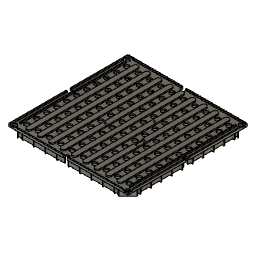
wordclock_Interior_Fusion360 (Autodesk Fusion 360 design; units mm, degrees)
Autodesk Fusion 360 part; units mm, degrees
note: some values were not read from the file. Chosen so that the rebuilt part matches the saved one: which bodies a step acts on.
(part 1 of 3)
sketch "Skizze1" plane through (0, 0, 0) normal (0, 0, 1) x (1, 0, 0)
  line L0 (0, 0) -> (204, 0)
  line L1 (204, 0) -> (204, 204)
  line L2 (204, 204) -> (0, 204)
  line L3 (0, 204) -> (0, 0)
  line L4 (2.15, 201.85) -> (201.85, 201.85)
  line L5 (201.85, 201.85) -> (201.85, 2.15)
  line L6 (201.85, 2.15) -> (2.15, 2.15)
  line L7 (2.15, 2.15) -> (2.15, 201.85)
  line L8 (93.75, 0) -> (100.25, 0)
  line L9 (100.25, 0) -> (100.25, 8.5)
  line L10 (100.25, 8.5) -> (93.75, 8.5)
  line L11 (93.75, 8.5) -> (93.75, 0)
  line L12 (93.75, 204) -> (100.25, 204)
  line L13 (100.25, 204) -> (100.25, 195.5)
  line L14 (100.25, 195.5) -> (93.75, 195.5)
  line L15 (93.75, 195.5) -> (93.75, 204)
  line L16 (0, 105.25) -> (8.5, 105.25)
  line L17 (8.5, 105.25) -> (8.5, 98.75)
  line L18 (8.5, 98.75) -> (0, 98.75)
  line L19 (0, 98.75) -> (0, 105.25)
  line L20 (204, 105.25) -> (195.5, 105.25)
  line L21 (195.5, 105.25) -> (195.5, 98.75)
  line L22 (195.5, 98.75) -> (204, 98.75)
  line L23 (204, 98.75) -> (204, 105.25)
  dimension "d1" = 204
  dimension "d2" = 204
  dimension "d3" = 2.15
  dimension "d4" = 2.15
  dimension "d5" = 2.15
  dimension "d6" = 2.15
  dimension "d387" = 8.5
  dimension "d388" = 6.5
  dimension "d389" = 93.75
  dimension "d390" = 8.5
  dimension "d391" = 6.5
  dimension "d392" = 93.75
  dimension "d397" = 8.5
  dimension "d398" = 6.5
  dimension "d399" = 98.75
  dimension "d415" = 6.5
  dimension "d416" = 8.5
  dimension "d417" = 98.75
  constraint horizontal L0
  constraint vertical L1
  constraint horizontal L2
  constraint vertical L3
  constraint coincident L0.start L3.end
  constraint horizontal L4
  constraint vertical L5
  constraint horizontal L6
  constraint vertical L7
  constraint horizontal L8
  constraint vertical L9
  constraint horizontal L10
  constraint vertical L11
  constraint coincident L0 L8.start
  constraint horizontal L12
  constraint vertical L13
  constraint horizontal L14
  constraint vertical L15
  constraint coincident L2 L12.start
  constraint horizontal L16
  constraint vertical L17
  constraint horizontal L18
  constraint vertical L19
  constraint coincident L3 L16.start
  constraint horizontal L20
  constraint vertical L21
  constraint horizontal L22
  constraint vertical L23
  constraint coincident L1 L20.start
  measures "d1" distance of L0.start L2.end
  measures "d2" distance of L1 L3
  measures "d3" distance of L2 L4
  measures "d4" distance of L1 L5
  measures "d5" distance of L0 L6
  measures "d6" distance of L3 L7
  measures "d387" distance of L8.start L10.end
  measures "d388" distance of L9.end L10.end
  measures "d389" distance of L3 L11
  measures "d390" distance of L12.start L14.end
  measures "d391" distance of L13.end L14.end
  measures "d392" distance of L3 L15
  measures "d397" distance of L16.start L16.end
  measures "d398" distance of L16.end L17.end
  measures "d399" distance of L0 L18
  measures "d415" distance of L20.end L21.end
  measures "d416" distance of L21.end L22.end
  measures "d417" distance of L0 L22
extrude "Extrusion1" add sketch "Skizze1" along normal blind 4 contours L6 L9 L10 L11 | L4 L5 L6 L7 L9 L10 L11 L13 L14 L15 L16 L17 L18 L20 L21 L22 | L7 L16 L17 L18 | L5 L20 L21 L22 | L4 L13 L14 L15 makes body 1
sketch "Skizze2" plane through (0, 0, 0) normal (0, 0, -1) x (1, 0, 0)
  line L0 (201.85, -2.15) -> (2.15, -2.15)
  line L1 (2.15, -2.15) -> (2.15, -201.85)
  line L2 (2.15, -201.85) -> (201.85, -201.85)
  line L3 (201.85, -201.85) -> (201.85, -2.15)
  line L4 (201.85, -18.65) -> (185.35, -2.15)
  line L5 (186.85, -2.15) -> (201.85, -17.15)
  line L6 (201.85, -201.85) -> (201.85, -2.15)
  line L7 (201.85, -2.15) -> (2.15, -2.15)
  line L8 (201.85, -186.85) -> (186.85, -201.85)
  line L9 (201.85, -185.35) -> (185.35, -201.85)
  line L10 (2.15, -186.85) -> (17.15, -201.85)
  line L11 (18.65, -201.85) -> (2.15, -185.35)
  line L12 (18.65, -2.15) -> (2.15, -18.65)
  line L13 (17.15, -2.15) -> (2.15, -17.15)
  point P0 (201.85, -201.85)
  point P1 (2.15, -201.85)
  point P2 (2.15, -2.15)
  point P3 (2.15, -2.15)
  dimension "d9" = 16.5
  dimension "d10" = 16.5
  dimension "d11" = 15
  dimension "d12" = 15
  dimension "d19" = 15
  dimension "d20" = 15
  dimension "d21" = 16.5
  dimension "d22" = 16.5
  dimension "d23" = 16.5
  dimension "d24" = 16.5
  dimension "d25" = 15
  dimension "d26" = 15
  dimension "d27" = 16.5
  dimension "d28" = 16.5
  dimension "d29" = 15
  dimension "d30" = 15
  constraint coincident L3 L4.start
  constraint coincident L0 L4.end
  constraint coincident L0 L5.start
  constraint coincident L3 L5.end
  constraint coincident L3 L8.start
  constraint coincident L2 L8.end
  constraint coincident L3 L9.start
  constraint coincident L2 L9.end
  constraint coincident L1 L10.start
  constraint coincident L2 L10.end
  constraint coincident L2 L11.start
  constraint coincident L1 L11.end
  constraint coincident L0 L12.start
  constraint coincident L1 L12.end
  constraint coincident L0 L13.start
  constraint coincident L1 L13.end
  constraint parallel L12 L13
  measures "d9" distance of L0.start L4.end
  measures "d10" distance of L0.start L4.start
  measures "d11" distance of L0.start L5.start
  measures "d12" distance of L0.start L5.end
  measures "d19" distance of P0 L8.start
  measures "d20" distance of P0 L8.end
  measures "d21" distance of L9.end P0
  measures "d22" distance of L9.start P0
  measures "d23" distance of P1 L11.end
  measures "d24" distance of P1 L11.start
  measures "d25" distance of L10.end P1
  measures "d26" distance of L10.start P1
  measures "d27" distance of L12.start P3
  measures "d28" distance of P3 L12.end
  measures "d29" distance of L13.end P3
  measures "d30" distance of L13.start P3
sketch "Skizze4" plane through (0, 0, 0) normal (0, 0, 1) x (1, 0, 0)
  line L0 (203.9938, 0) -> (0, 0)
  line L1 (0, 203.9937) -> (0, 0)
  line L2 (0, 0) -> (203.9938, 0)
  line L3 (203.9938, 0) -> (203.9938, 203.9937)
  line L4 (203.9938, 203.9937) -> (0, 203.9937)
  line L5 (21.7426, 192.1915) -> (21.7426, 185.9421)
  line L6 (21.7426, 185.9421) -> (20.443, 185.9421)
  line L7 (20.443, 185.9421) -> (20.443, 190.5017)
  line L8 (20.443, 190.5017) -> (17.8837, 190.5017)
  line L9 (17.8837, 190.5017) -> (17.8837, 186.7579)
  line L10 (17.8837, 186.7579) -> (16.5841, 186.7579)
  line L11 (16.5841, 186.7579) -> (16.5841, 190.5017)
  line L12 (16.5841, 190.5017) -> (14.3696, 190.5017)
  line L13 (14.3696, 190.5017) -> (14.3696, 186.0878)
  line L14 (14.3696, 186.0878) -> (13.07, 186.0878)
  line L15 (13.07, 186.0878) -> (13.07, 192.1915)
  line L16 (13.07, 192.1915) -> (21.7426, 192.1915)
  spline S0 degree 3 poles (21.9017, 171.8232) (21.9017, 169.609) (20.7348, 168.298) (19.3291, 168.298) knots 0 0 0 0 1 1 1 1
  spline S1 degree 3 poles (19.3291, 168.298) (18.0693, 168.298) (17.4196, 169.1574) (16.9819, 170.3665) knots 0 0 0 0 1 1 1 1
  line L17 (16.9819, 170.3665) -> (16.4913, 171.6193)
  spline S2 degree 3 poles (16.4913, 171.6193) (16.1863, 172.4788) (15.9343, 173.2508) (15.2713, 173.2508) knots 0 0 0 0 1 1 1 1
  spline S3 degree 3 poles (15.2713, 173.2508) (14.6215, 173.2508) (14.2502, 172.639) (14.2502, 171.7358) knots 0 0 0 0 1 1 1 1
  spline S4 degree 3 poles (14.2502, 171.7358) (14.2502, 170.7744) (14.5287, 170.1043) (14.9928, 169.4633) knots 0 0 0 0 1 1 1 1
  line L18 (14.9928, 169.4633) -> (14.0115, 168.5893)
  spline S5 degree 3 poles (14.0115, 168.5893) (13.3352, 169.3759) (12.9109, 170.483) (12.9109, 171.6484) knots 0 0 0 0 1 1 1 1
  spline S6 degree 3 poles (12.9109, 171.6484) (12.9109, 173.5859) (13.9717, 174.9552) (15.3509, 174.9552) knots 0 0 0 0 1 1 1 1
  spline S7 degree 3 poles (15.3509, 174.9552) (16.6239, 174.9552) (17.3002, 173.9209) (17.6583, 172.9158) knots 0 0 0 0 1 1 1 1
  line L19 (17.6583, 172.9158) -> (18.1754, 171.6193)
  spline S8 degree 3 poles (18.1754, 171.6193) (18.5335, 170.6724) (18.7456, 170.0169) (19.5148, 170.0169) knots 0 0 0 0 1 1 1 1
  spline S9 degree 3 poles (19.5148, 170.0169) (20.1248, 170.0169) (20.5624, 170.6142) (20.5624, 171.7213) knots 0 0 0 0 1 1 1 1
  spline S10 degree 3 poles (20.5624, 171.7213) (20.5624, 172.7264) (20.1646, 173.6733) (19.5811, 174.3871) knots 0 0 0 0 1 1 1 1
  line L20 (19.5811, 174.3871) -> (20.6287, 175.3777)
  spline S11 degree 3 poles (20.6287, 175.3777) (21.4376, 174.4308) (21.9017, 173.1634) (21.9017, 171.8232) knots 0 0 0 0 1 1 1 1
  line L21 (21.7426, 157.5587) -> (21.7426, 155.8397)
  line L22 (21.7426, 155.8397) -> (19.1833, 155.8397)
  line L23 (19.1833, 155.8397) -> (17.6185, 154.485)
  line L24 (17.6185, 154.485) -> (21.7426, 152.0814)
  line L25 (21.7426, 152.0814) -> (21.7426, 150.2022)
  line L26 (21.7426, 150.2022) -> (16.4383, 153.4507)
  line L27 (16.4383, 153.4507) -> (13.07, 150.5081)
  line L28 (13.07, 150.5081) -> (13.07, 152.4019)
  line L29 (13.07, 152.4019) -> (17.0085, 155.796)
  line L30 (17.0085, 155.796) -> (17.0085, 155.8398)
  line L31 (17.0085, 155.8398) -> (13.07, 155.8398)
  line L32 (13.07, 155.8398) -> (13.07, 157.5587)
  line L33 (13.07, 157.5587) -> (21.7426, 157.5587)
  line L34 (21.7426, 140.0602) -> (21.7426, 133.7672)
  line L35 (21.7426, 133.7672) -> (20.443, 133.7672)
  line L36 (20.443, 133.7672) -> (20.443, 136.0688)
  line L37 (20.443, 136.0688) -> (14.3696, 136.0688)
  line L38 (14.3696, 136.0688) -> (14.3696, 133.7672)
  line L39 (14.3696, 133.7672) -> (13.07, 133.7672)
  line L40 (13.07, 133.7672) -> (13.07, 140.0602)
  line L41 (13.07, 140.0602) -> (14.3696, 140.0602)
  line L42 (14.3696, 140.0602) -> (14.3696, 137.7586)
  line L43 (14.3696, 137.7586) -> (20.443, 137.7586)
  line L44 (20.443, 137.7586) -> (20.443, 140.0602)
  line L45 (20.443, 140.0602) -> (21.7426, 140.0602)
  spline S12 degree 3 poles (21.9017, 119.4152) (21.9017, 117.201) (20.7348, 115.8899) (19.3291, 115.8899) knots 0 0 0 0 1 1 1 1
  spline S13 degree 3 poles (19.3291, 115.8899) (18.0693, 115.8899) (17.4196, 116.7494) (16.9819, 117.9585) knots 0 0 0 0 1 1 1 1
  line L46 (16.9819, 117.9585) -> (16.4913, 119.2113)
  spline S14 degree 3 poles (16.4913, 119.2113) (16.1863, 120.0707) (15.9343, 120.8428) (15.2713, 120.8428) knots 0 0 0 0 1 1 1 1
  spline S15 degree 3 poles (15.2713, 120.8428) (14.6215, 120.8428) (14.2502, 120.231) (14.2502, 119.3278) knots 0 0 0 0 1 1 1 1
  spline S16 degree 3 poles (14.2502, 119.3278) (14.2502, 118.3664) (14.5287, 117.6963) (14.9928, 117.0553) knots 0 0 0 0 1 1 1 1
  line L47 (14.9928, 117.0553) -> (14.0115, 116.1813)
  spline S17 degree 3 poles (14.0115, 116.1813) (13.3352, 116.9679) (12.9109, 118.075) (12.9109, 119.2404) knots 0 0 0 0 1 1 1 1
  spline S18 degree 3 poles (12.9109, 119.2404) (12.9109, 121.1779) (13.9717, 122.5472) (15.3509, 122.5472) knots 0 0 0 0 1 1 1 1
  spline S19 degree 3 poles (15.3509, 122.5472) (16.6239, 122.5472) (17.3002, 121.5129) (17.6583, 120.5078) knots 0 0 0 0 1 1 1 1
  line L48 (17.6583, 120.5078) -> (18.1754, 119.2113)
  spline S20 degree 3 poles (18.1754, 119.2113) (18.5335, 118.2644) (18.7456, 117.6089) (19.5148, 117.6089) knots 0 0 0 0 1 1 1 1
  spline S21 degree 3 poles (19.5148, 117.6089) (20.1248, 117.6089) (20.5624, 118.2061) (20.5624, 119.3133) knots 0 0 0 0 1 1 1 1
  spline S22 degree 3 poles (20.5624, 119.3133) (20.5624, 120.3184) (20.1646, 121.2653) (19.5811, 121.9791) knots 0 0 0 0 1 1 1 1
  line L49 (19.5811, 121.9791) -> (20.6287, 122.9696)
  spline S23 degree 3 poles (20.6287, 122.9696) (21.4376, 122.0228) (21.9017, 120.7554) (21.9017, 119.4152) knots 0 0 0 0 1 1 1 1
  line L50 (21.7426, 102.8199) -> (21.7426, 101.1301)
  line L51 (21.7426, 101.1301) -> (14.3696, 101.1301)
  line L52 (14.3696, 101.1301) -> (14.3696, 98.1292)
  line L53 (14.3696, 98.1292) -> (13.07, 98.1292)
  line L54 (13.07, 98.1292) -> (13.07, 105.8207)
  line L55 (13.07, 105.8207) -> (14.3696, 105.8207)
  line L56 (14.3696, 105.8207) -> (14.3696, 102.8199)
  line L57 (14.3696, 102.8199) -> (21.7426, 102.8199)
  spline S24 degree 3 poles (17.1278, 85.4088) (16.2128, 85.1175) (15.2315, 84.8261) (14.2635, 84.5639) knots 0 0 0 0 1 1 1 1
  line L58 (14.2635, 84.5639) -> (14.2635, 84.5056)
  spline S25 degree 3 poles (14.2635, 84.5056) (15.2315, 84.2434) (16.2128, 83.9375) (17.1278, 83.6607) knots 0 0 0 0 1 1 1 1
  line L59 (17.1278, 83.6607) -> (18.1887, 83.3257)
  line L60 (18.1887, 83.3257) -> (18.1887, 85.7439)
  line L61 (18.1887, 85.7439) -> (17.1278, 85.4088)
  line L62 (21.7426, 88.5845) -> (21.7426, 86.8655)
  line L63 (21.7426, 86.8655) -> (19.3954, 86.1226)
  line L64 (19.3954, 86.1226) -> (19.3954, 82.9469)
  line L65 (19.3954, 82.9469) -> (21.7426, 82.2186)
  line L66 (21.7426, 82.2186) -> (21.7426, 80.4268)
  line L67 (21.7426, 80.4268) -> (13.07, 83.5151)
  line L68 (13.07, 83.5151) -> (13.07, 85.4962)
  line L69 (13.07, 85.4962) -> (21.7426, 88.5845)
  line L70 (21.7426, 69.673) -> (21.7426, 67.9832)
  line L71 (21.7426, 67.9832) -> (18.1224, 67.9832)
  line L72 (18.1224, 67.9832) -> (18.1224, 64.2394)
  line L73 (18.1224, 64.2394) -> (16.8228, 64.2394)
  line L74 (16.8228, 64.2394) -> (16.8228, 67.9832)
  line L75 (16.8228, 67.9832) -> (14.3696, 67.9832)
  line L76 (14.3696, 67.9832) -> (14.3696, 63.5839)
  line L77 (14.3696, 63.5839) -> (13.07, 63.5839)
  line L78 (13.07, 63.5839) -> (13.07, 69.673)
  line L79 (13.07, 69.673) -> (21.7426, 69.673)
  spline S26 degree 3 poles (21.9017, 49.5524) (21.9017, 47.4547) (20.8011, 46.2456) (18.4274, 46.2456) knots 0 0 0 0 1 1 1 1
  line L80 (18.4274, 46.2456) -> (13.07, 46.2456)
  line L81 (13.07, 46.2456) -> (13.07, 47.8626)
  line L82 (13.07, 47.8626) -> (18.5467, 47.8626)
  spline S27 degree 3 poles (18.5467, 47.8626) (19.9656, 47.8626) (20.5624, 48.5181) (20.5624, 49.5524) knots 0 0 0 0 1 1 1 1
  spline S28 degree 3 poles (20.5624, 49.5524) (20.5624, 50.5721) (19.9656, 51.1985) (18.5467, 51.1985) knots 0 0 0 0 1 1 1 1
  line L83 (18.5467, 51.1985) -> (13.07, 51.1985)
  line L84 (13.07, 51.1985) -> (13.07, 52.8883)
  line L85 (13.07, 52.8883) -> (18.4274, 52.8883)
  spline S29 degree 3 poles (18.4274, 52.8883) (20.8011, 52.8883) (21.9017, 51.6355) (21.9017, 49.5524) knots 0 0 0 0 1 1 1 1
  spline S30 degree 3 poles (12.3539, 51.0382) (12.3539, 50.5138) (12.0091, 50.1351) (11.5317, 50.1351) knots 0 0 0 0 1 1 1 1
  spline S31 degree 3 poles (11.5317, 50.1351) (11.0544, 50.1351) (10.7096, 50.5138) (10.7096, 51.0382) knots 0 0 0 0 1 1 1 1
  spline S32 degree 3 poles (10.7096, 51.0382) (10.7096, 51.5627) (11.0544, 51.9414) (11.5317, 51.9414) knots 0 0 0 0 1 1 1 1
  spline S33 degree 3 poles (11.5317, 51.9414) (12.0091, 51.9414) (12.3539, 51.5627) (12.3539, 51.0382) knots 0 0 0 0 1 1 1 1
  spline S34 degree 3 poles (12.3539, 48.0956) (12.3539, 47.5712) (12.0091, 47.1925) (11.5317, 47.1925) knots 0 0 0 0 1 1 1 1
  spline S35 degree 3 poles (11.5317, 47.1925) (11.0544, 47.1925) (10.7096, 47.5712) (10.7096, 48.0956) knots 0 0 0 0 1 1 1 1
  spline S36 degree 3 poles (10.7096, 48.0956) (10.7096, 48.6201) (11.0544, 48.9988) (11.5317, 48.9988) knots 0 0 0 0 1 1 1 1
  spline S37 degree 3 poles (11.5317, 48.9988) (12.0091, 48.9988) (12.3539, 48.6201) (12.3539, 48.0956) knots 0 0 0 0 1 1 1 1
  line L86 (21.7426, 35.3898) -> (21.7426, 33.7728)
  line L87 (21.7426, 33.7728) -> (17.95, 33.7728)
  spline S38 degree 3 poles (17.95, 33.7728) (16.9819, 33.7728) (15.9476, 33.9331) (15.0194, 34.0059) knots 0 0 0 0 1 1 1 1
  line L88 (15.0194, 34.0059) -> (15.0194, 33.9622)
  line L89 (15.0194, 33.9622) -> (16.8626, 33.1027)
  line L90 (16.8626, 33.1027) -> (21.7426, 30.5826)
  line L91 (21.7426, 30.5826) -> (21.7426, 28.8054)
  line L92 (21.7426, 28.8054) -> (13.07, 28.8054)
  line L93 (13.07, 28.8054) -> (13.07, 30.4224)
  line L94 (13.07, 30.4224) -> (16.8361, 30.4224)
  spline S39 degree 3 poles (16.8361, 30.4224) (17.8041, 30.4224) (18.9048, 30.2621) (19.7932, 30.1893) knots 0 0 0 0 1 1 1 1
  line L95 (19.7932, 30.1893) -> (19.7932, 30.233)
  line L96 (19.7932, 30.233) -> (17.9367, 31.0925)
  line L97 (17.9367, 31.0925) -> (13.07, 33.6126)
  line L98 (13.07, 33.6126) -> (13.07, 35.3898)
  line L99 (13.07, 35.3898) -> (21.7426, 35.3898)
  line L100 (21.7426, 17.2649) -> (21.7426, 15.5751)
  line L101 (21.7426, 15.5751) -> (18.1224, 15.5751)
  line L102 (18.1224, 15.5751) -> (18.1224, 11.8313)
  line L103 (18.1224, 11.8313) -> (16.8228, 11.8313)
  line L104 (16.8228, 11.8313) -> (16.8228, 15.5751)
  line L105 (16.8228, 15.5751) -> (14.3696, 15.5751)
  line L106 (14.3696, 15.5751) -> (14.3696, 11.1758)
  line L107 (14.3696, 11.1758) -> (13.07, 11.1758)
  line L108 (13.07, 11.1758) -> (13.07, 17.2649)
  line L109 (13.07, 17.2649) -> (21.7426, 17.2649)
  line L110 (40.7851, 192.8033) -> (40.7851, 185.7819)
  line L111 (40.7851, 185.7819) -> (39.4855, 185.7819)
  line L112 (39.4855, 185.7819) -> (39.4855, 190.7347)
  line L113 (39.4855, 190.7347) -> (33.0408, 185.8401)
  line L114 (33.0408, 185.8401) -> (32.1125, 185.8401)
  line L115 (32.1125, 185.8401) -> (32.1125, 192.3663)
  line L116 (32.1125, 192.3663) -> (33.3988, 192.3663)
  line L117 (33.3988, 192.3663) -> (33.3988, 187.9232)
  line L118 (33.3988, 187.9232) -> (39.8568, 192.8033)
  line L119 (39.8568, 192.8033) -> (40.7851, 192.8033)
  line L120 (40.7851, 174.7221) -> (40.7851, 168.4728)
  line L121 (40.7851, 168.4728) -> (39.4855, 168.4728)
  line L122 (39.4855, 168.4728) -> (39.4855, 173.0323)
  line L123 (39.4855, 173.0323) -> (36.9262, 173.0323)
  line L124 (36.9262, 173.0323) -> (36.9262, 169.2885)
  line L125 (36.9262, 169.2885) -> (35.6266, 169.2885)
  line L126 (35.6266, 169.2885) -> (35.6266, 173.0323)
  line L127 (35.6266, 173.0323) -> (33.4121, 173.0323)
  line L128 (33.4121, 173.0323) -> (33.4121, 168.6184)
  line L129 (33.4121, 168.6184) -> (32.1125, 168.6184)
  line L130 (32.1125, 168.6184) -> (32.1125, 174.7221)
  line L131 (32.1125, 174.7221) -> (40.7851, 174.7221)
  line L132 (40.7851, 157.7044) -> (40.7851, 156.0146)
  line L133 (40.7851, 156.0146) -> (36.9394, 156.0146)
  line L134 (36.9394, 156.0146) -> (36.9394, 152.7515)
  line L135 (36.9394, 152.7515) -> (40.7851, 152.7515)
  line L136 (40.7851, 152.7515) -> (40.7851, 151.0617)
  line L137 (40.7851, 151.0617) -> (32.1125, 151.0617)
  line L138 (32.1125, 151.0617) -> (32.1125, 152.7515)
  line L139 (32.1125, 152.7515) -> (35.6001, 152.7515)
  line L140 (35.6001, 152.7515) -> (35.6001, 156.0146)
  line L141 (35.6001, 156.0146) -> (32.1125, 156.0146)
  line L142 (32.1125, 156.0146) -> (32.1125, 157.7044)
  line L143 (32.1125, 157.7044) -> (40.7851, 157.7044)
  line L144 (40.7851, 140.2059) -> (40.7851, 138.5889)
  line L145 (40.7851, 138.5889) -> (36.9925, 138.5889)
  spline S40 degree 3 poles (36.9925, 138.5889) (36.0244, 138.5889) (34.9901, 138.7492) (34.0618, 138.822) knots 0 0 0 0 1 1 1 1
  line L146 (34.0618, 138.822) -> (34.0618, 138.7783)
  line L147 (34.0618, 138.7783) -> (35.9051, 137.9188)
  line L148 (35.9051, 137.9188) -> (40.7851, 135.3987)
  line L149 (40.7851, 135.3987) -> (40.7851, 133.6215)
  line L150 (40.7851, 133.6215) -> (32.1125, 133.6215)
  line L151 (32.1125, 133.6215) -> (32.1125, 135.2384)
  line L152 (32.1125, 135.2384) -> (35.8786, 135.2384)
  spline S41 degree 3 poles (35.8786, 135.2384) (36.8466, 135.2384) (37.9473, 135.0782) (38.8357, 135.0054) knots 0 0 0 0 1 1 1 1
  line L153 (38.8357, 135.0054) -> (38.8357, 135.0491)
  line L154 (38.8357, 135.0491) -> (36.9792, 135.9085)
  line L155 (36.9792, 135.9085) -> (32.1125, 138.4287)
  line L156 (32.1125, 138.4287) -> (32.1125, 140.2059)
  line L157 (32.1125, 140.2059) -> (40.7851, 140.2059)
  line L158 (40.7851, 122.9259) -> (40.7851, 115.9045)
  line L159 (40.7851, 115.9045) -> (39.4855, 115.9045)
  line L160 (39.4855, 115.9045) -> (39.4855, 120.8574)
  line L161 (39.4855, 120.8574) -> (33.0408, 115.9628)
  line L162 (33.0408, 115.9628) -> (32.1125, 115.9628)
  line L163 (32.1125, 115.9628) -> (32.1125, 122.4889)
  line L164 (32.1125, 122.4889) -> (33.3988, 122.4889)
  line L165 (33.3988, 122.4889) -> (33.3988, 118.0459)
  line L166 (33.3988, 118.0459) -> (39.8568, 122.9259)
  line L167 (39.8568, 122.9259) -> (40.7851, 122.9259)
  line L168 (40.7851, 104.8884) -> (40.7851, 103.0093)
  line L169 (40.7851, 103.0093) -> (37.7086, 102.2809)
  spline S42 degree 3 poles (37.7086, 102.2809) (37.1649, 102.1498) (36.6212, 102.077) (36.0907, 101.9895) knots 0 0 0 0 1 1 1 1
  line L170 (36.0907, 101.9895) -> (36.0907, 101.9458)
  spline S43 degree 3 poles (36.0907, 101.9458) (36.6212, 101.8876) (37.1649, 101.771) (37.7086, 101.6399) knots 0 0 0 0 1 1 1 1
  line L171 (37.7086, 101.6399) -> (40.7851, 100.897)
  line L172 (40.7851, 100.897) -> (40.7851, 98.9887)
  line L173 (40.7851, 98.9887) -> (32.1125, 97.7067)
  line L174 (32.1125, 97.7067) -> (32.1125, 99.4111)
  line L175 (32.1125, 99.4111) -> (37.1383, 99.8773)
  spline S44 degree 3 poles (37.1383, 99.8773) (37.8544, 99.9355) (38.3981, 99.9501) (39.2203, 99.9938) knots 0 0 0 0 1 1 1 1
  line L176 (39.2203, 99.9938) -> (39.2203, 100.0521)
  spline S45 degree 3 poles (39.2203, 100.0521) (38.3981, 100.1978) (37.8544, 100.3289) (37.1383, 100.5182) knots 0 0 0 0 1 1 1 1
  line L177 (37.1383, 100.5182) -> (34.327, 101.2612)
  line L178 (34.327, 101.2612) -> (34.327, 102.5285)
  line L179 (34.327, 102.5285) -> (37.1383, 103.3152)
  spline S46 degree 3 poles (37.1383, 103.3152) (37.8677, 103.49) (38.4114, 103.6211) (39.2203, 103.7813) knots 0 0 0 0 1 1 1 1
  line L180 (39.2203, 103.7813) -> (39.2203, 103.825)
  spline S47 degree 3 poles (39.2203, 103.825) (38.4114, 103.8541) (37.8677, 103.8978) (37.1383, 103.9561) knots 0 0 0 0 1 1 1 1
  line L181 (37.1383, 103.9561) -> (32.1125, 104.4368)
  line L182 (32.1125, 104.4368) -> (32.1125, 106.2432)
  line L183 (32.1125, 106.2432) -> (40.7851, 104.8884)
  spline S48 degree 3 poles (36.1703, 85.4088) (35.2553, 85.1175) (34.274, 84.8261) (33.306, 84.5639) knots 0 0 0 0 1 1 1 1
  line L184 (33.306, 84.5639) -> (33.306, 84.5056)
  spline S49 degree 3 poles (33.306, 84.5056) (34.274, 84.2434) (35.2553, 83.9375) (36.1703, 83.6607) knots 0 0 0 0 1 1 1 1
  line L185 (36.1703, 83.6607) -> (37.2312, 83.3257)
  line L186 (37.2312, 83.3257) -> (37.2312, 85.7439)
  line L187 (37.2312, 85.7439) -> (36.1703, 85.4088)
  line L188 (40.7851, 88.5845) -> (40.7851, 86.8655)
  line L189 (40.7851, 86.8655) -> (38.4379, 86.1226)
  line L190 (38.4379, 86.1226) -> (38.4379, 82.9469)
  line L191 (38.4379, 82.9469) -> (40.7851, 82.2186)
  line L192 (40.7851, 82.2186) -> (40.7851, 80.4268)
  line L193 (40.7851, 80.4268) -> (32.1125, 83.5151)
  line L194 (32.1125, 83.5151) -> (32.1125, 85.4962)
  line L195 (32.1125, 85.4962) -> (40.7851, 88.5845)
  line L196 (40.7851, 70.3285) -> (40.7851, 68.7116)
  line L197 (40.7851, 68.7116) -> (36.9925, 68.7116)
  spline S50 degree 3 poles (36.9925, 68.7116) (36.0244, 68.7116) (34.9901, 68.8718) (34.0618, 68.9446) knots 0 0 0 0 1 1 1 1
  line L198 (34.0618, 68.9446) -> (34.0618, 68.9009)
  line L199 (34.0618, 68.9009) -> (35.9051, 68.0415)
  line L200 (35.9051, 68.0415) -> (40.7851, 65.5213)
  line L201 (40.7851, 65.5213) -> (40.7851, 63.7441)
  line L202 (40.7851, 63.7441) -> (32.1125, 63.7441)
  line L203 (32.1125, 63.7441) -> (32.1125, 65.3611)
  line L204 (32.1125, 65.3611) -> (35.8786, 65.3611)
  spline S51 degree 3 poles (35.8786, 65.3611) (36.8466, 65.3611) (37.9473, 65.2008) (38.8357, 65.128) knots 0 0 0 0 1 1 1 1
  line L205 (38.8357, 65.128) -> (38.8357, 65.1717)
  line L206 (38.8357, 65.1717) -> (36.9792, 66.0312)
  line L207 (36.9792, 66.0312) -> (32.1125, 68.5513)
  line L208 (32.1125, 68.5513) -> (32.1125, 70.3285)
  line L209 (32.1125, 70.3285) -> (40.7851, 70.3285)
  line L210 (40.7851, 53.0485) -> (40.7851, 46.0271)
  line L211 (40.7851, 46.0271) -> (39.4855, 46.0271)
  line L212 (39.4855, 46.0271) -> (39.4855, 50.98)
  line L213 (39.4855, 50.98) -> (33.0408, 46.0854)
  line L214 (33.0408, 46.0854) -> (32.1125, 46.0854)
  line L215 (32.1125, 46.0854) -> (32.1125, 52.6115)
  line L216 (32.1125, 52.6115) -> (33.3988, 52.6115)
  line L217 (33.3988, 52.6115) -> (33.3988, 48.1685)
  line L218 (33.3988, 48.1685) -> (39.8568, 53.0485)
  line L219 (39.8568, 53.0485) -> (40.7851, 53.0485)
  line L220 (40.7851, 35.2441) -> (40.7851, 28.9511)
  line L221 (40.7851, 28.9511) -> (39.4855, 28.9511)
  line L222 (39.4855, 28.9511) -> (39.4855, 31.2527)
  line L223 (39.4855, 31.2527) -> (33.4121, 31.2527)
  line L224 (33.4121, 31.2527) -> (33.4121, 28.9511)
  line L225 (33.4121, 28.9511) -> (32.1125, 28.9511)
  line L226 (32.1125, 28.9511) -> (32.1125, 35.2441)
  line L227 (32.1125, 35.2441) -> (33.4121, 35.2441)
  line L228 (33.4121, 35.2441) -> (33.4121, 32.9425)
  line L229 (33.4121, 32.9425) -> (39.4855, 32.9425)
  line L230 (39.4855, 32.9425) -> (39.4855, 35.2441)
  line L231 (39.4855, 35.2441) -> (40.7851, 35.2441)
  spline S52 degree 3 poles (40.9442, 14.0456) (40.9442, 12.8219) (40.4668, 11.7439) (39.9099, 11.1321) knots 0 0 0 0 1 1 1 1
  line L232 (39.9099, 11.1321) -> (36.0907, 11.1321)
  line L233 (36.0907, 11.1321) -> (36.0907, 14.3078)
  line L234 (36.0907, 14.3078) -> (37.3505, 14.3078)
  line L235 (37.3505, 14.3078) -> (37.3505, 12.6617)
  line L236 (37.3505, 12.6617) -> (39.2203, 12.6617)
  spline S53 degree 3 poles (39.2203, 12.6617) (39.4723, 12.9385) (39.6049, 13.4338) (39.6049, 13.9436) knots 0 0 0 0 1 1 1 1
  spline S54 degree 3 poles (39.6049, 13.9436) (39.6049, 15.6334) (38.4114, 16.5511) (36.4355, 16.5511) knots 0 0 0 0 1 1 1 1
  spline S55 degree 3 poles (36.4355, 16.5511) (34.4862, 16.5511) (33.2927, 15.4877) (33.2927, 13.9728) knots 0 0 0 0 1 1 1 1
  spline S56 degree 3 poles (33.2927, 13.9728) (33.2927, 13.1424) (33.5844, 12.6471) (33.9955, 12.2101) knots 0 0 0 0 1 1 1 1
  line L237 (33.9955, 12.2101) -> (33.0408, 11.2778)
  spline S57 degree 3 poles (33.0408, 11.2778) (32.4971, 11.8459) (31.9534, 12.7054) (31.9534, 13.9728) knots 0 0 0 0 1 1 1 1
  spline S58 degree 3 poles (31.9534, 13.9728) (31.9534, 16.4492) (33.6242, 18.2992) (36.4753, 18.2992) knots 0 0 0 0 1 1 1 1
  spline S59 degree 3 poles (36.4753, 18.2992) (39.3529, 18.2992) (40.9442, 16.4637) (40.9442, 14.0456) knots 0 0 0 0 1 1 1 1
  line L238 (59.8276, 192.5556) -> (59.8276, 189.9627)
  spline S60 degree 3 poles (59.8276, 189.9627) (59.8276, 187.2386) (58.3291, 185.5634) (55.4515, 185.5634) knots 0 0 0 0 1 1 1 1
  spline S61 degree 3 poles (55.4515, 185.5634) (52.5872, 185.5634) (51.155, 187.2386) (51.155, 190.0501) knots 0 0 0 0 1 1 1 1
  line L239 (51.155, 190.0501) -> (51.155, 192.5556)
  line L240 (51.155, 192.5556) -> (59.8276, 192.5556)
  line L241 (58.5811, 190.8658) -> (52.4015, 190.8658)
  line L242 (52.4015, 190.8658) -> (52.4015, 190.152)
  spline S62 degree 3 poles (52.4015, 190.152) (52.4015, 188.3311) (53.3298, 187.2969) (55.4515, 187.2969) knots 0 0 0 0 1 1 1 1
  spline S63 degree 3 poles (55.4515, 187.2969) (57.5865, 187.2969) (58.5811, 188.3311) (58.5811, 190.152) knots 0 0 0 0 1 1 1 1
  line L243 (58.5811, 190.152) -> (58.5811, 190.8658)
  line L244 (59.8276, 174.9989) -> (59.8276, 173.3091)
  line L245 (59.8276, 173.3091) -> (56.4328, 173.3091)
  line L246 (56.4328, 173.3091) -> (56.4328, 171.8815)
  line L247 (56.4328, 171.8815) -> (59.8276, 169.8421)
  line L248 (59.8276, 169.8421) -> (59.8276, 167.9338)
  line L249 (59.8276, 167.9338) -> (56.2074, 170.2063)
  spline S64 degree 3 poles (56.2074, 170.2063) (55.8493, 169.07) (55.0404, 168.3125) (53.7276, 168.3125) knots 0 0 0 0 1 1 1 1
  spline S65 degree 3 poles (53.7276, 168.3125) (51.7915, 168.3125) (51.155, 169.8421) (51.155, 171.8232) knots 0 0 0 0 1 1 1 1
  line L250 (51.155, 171.8232) -> (51.155, 174.9989)
  line L251 (51.155, 174.9989) -> (59.8276, 174.9989)
  line L252 (55.2128, 173.3091) -> (52.3883, 173.3091)
  line L253 (52.3883, 173.3091) -> (52.3883, 171.998)
  spline S66 degree 3 poles (52.3883, 171.998) (52.3883, 170.687) (52.733, 169.9732) (53.7276, 169.9732) knots 0 0 0 0 1 1 1 1
  spline S67 degree 3 poles (53.7276, 169.9732) (54.7089, 169.9732) (55.2128, 170.687) (55.2128, 171.998) knots 0 0 0 0 1 1 1 1
  line L254 (55.2128, 171.998) -> (55.2128, 173.3091)
  line L255 (59.8276, 157.2528) -> (59.8276, 151.0034)
  line L256 (59.8276, 151.0034) -> (58.528, 151.0034)
  line L257 (58.528, 151.0034) -> (58.528, 155.563)
  line L258 (58.528, 155.563) -> (55.9687, 155.563)
  line L259 (55.9687, 155.563) -> (55.9687, 151.8192)
  line L260 (55.9687, 151.8192) -> (54.6691, 151.8192)
  line L261 (54.6691, 151.8192) -> (54.6691, 155.563)
  line L262 (54.6691, 155.563) -> (52.4545, 155.563)
  line L263 (52.4545, 155.563) -> (52.4545, 151.1491)
  line L264 (52.4545, 151.1491) -> (51.155, 151.1491)
  line L265 (51.155, 151.1491) -> (51.155, 157.2528)
  line L266 (51.155, 157.2528) -> (59.8276, 157.2528)
  line L267 (59.8276, 140.0602) -> (59.8276, 133.7672)
  line L268 (59.8276, 133.7672) -> (58.528, 133.7672)
  line L269 (58.528, 133.7672) -> (58.528, 136.0688)
  line L270 (58.528, 136.0688) -> (52.4545, 136.0688)
  line L271 (52.4545, 136.0688) -> (52.4545, 133.7672)
  line L272 (52.4545, 133.7672) -> (51.155, 133.7672)
  line L273 (51.155, 133.7672) -> (51.155, 140.0602)
  line L274 (51.155, 140.0602) -> (52.4545, 140.0602)
  line L275 (52.4545, 140.0602) -> (52.4545, 137.7586)
  line L276 (52.4545, 137.7586) -> (58.528, 137.7586)
  line L277 (58.528, 137.7586) -> (58.528, 140.0602)
  line L278 (58.528, 140.0602) -> (59.8276, 140.0602)
  line L279 (59.8276, 120.4349) -> (59.8276, 118.4392)
  line L280 (59.8276, 118.4392) -> (51.155, 115.482)
  line L281 (51.155, 115.482) -> (51.155, 117.2155)
  line L282 (51.155, 117.2155) -> (55.5178, 118.5412)
  spline S68 degree 3 poles (55.5178, 118.5412) (56.4991, 118.8325) (57.3478, 119.051) (58.3424, 119.3715) knots 0 0 0 0 1 1 1 1
  line L283 (58.3424, 119.3715) -> (58.3424, 119.4298)
  spline S69 degree 3 poles (58.3424, 119.4298) (57.3478, 119.7502) (56.4991, 119.9688) (55.5178, 120.2747) knots 0 0 0 0 1 1 1 1
  line L284 (55.5178, 120.2747) -> (51.155, 121.6149)
  line L285 (51.155, 121.6149) -> (51.155, 123.4066)
  line L286 (51.155, 123.4066) -> (59.8276, 120.4349)
  line L287 (59.8276, 105.1215) -> (59.8276, 98.8285)
  line L288 (59.8276, 98.8285) -> (58.528, 98.8285)
  line L289 (58.528, 98.8285) -> (58.528, 101.1301)
  line L290 (58.528, 101.1301) -> (52.4545, 101.1301)
  line L291 (52.4545, 101.1301) -> (52.4545, 98.8285)
  line L292 (52.4545, 98.8285) -> (51.155, 98.8285)
  line L293 (51.155, 98.8285) -> (51.155, 105.1215)
  line L294 (51.155, 105.1215) -> (52.4545, 105.1215)
  line L295 (52.4545, 105.1215) -> (52.4545, 102.8199)
  line L296 (52.4545, 102.8199) -> (58.528, 102.8199)
  line L297 (58.528, 102.8199) -> (58.528, 105.1215)
  line L298 (58.528, 105.1215) -> (59.8276, 105.1215)
  line L299 (59.8276, 87.3754) -> (59.8276, 81.1261)
  line L300 (59.8276, 81.1261) -> (58.528, 81.1261)
  line L301 (58.528, 81.1261) -> (58.528, 85.6856)
  line L302 (58.528, 85.6856) -> (55.9687, 85.6856)
  line L303 (55.9687, 85.6856) -> (55.9687, 81.9418)
  line L304 (55.9687, 81.9418) -> (54.6691, 81.9418)
  line L305 (54.6691, 81.9418) -> (54.6691, 85.6856)
  line L306 (54.6691, 85.6856) -> (52.4545, 85.6856)
  line L307 (52.4545, 85.6856) -> (52.4545, 81.2717)
  line L308 (52.4545, 81.2717) -> (51.155, 81.2717)
  line L309 (51.155, 81.2717) -> (51.155, 87.3754)
  line L310 (51.155, 87.3754) -> (59.8276, 87.3754)
  line L311 (59.8276, 70.1828) -> (59.8276, 68.493)
  line L312 (59.8276, 68.493) -> (56.4328, 68.493)
  line L313 (56.4328, 68.493) -> (56.4328, 67.0655)
  line L314 (56.4328, 67.0655) -> (59.8276, 65.026)
  line L315 (59.8276, 65.026) -> (59.8276, 63.1177)
  line L316 (59.8276, 63.1177) -> (56.2074, 65.3902)
  spline S70 degree 3 poles (56.2074, 65.3902) (55.8493, 64.254) (55.0404, 63.4965) (53.7276, 63.4965) knots 0 0 0 0 1 1 1 1
  spline S71 degree 3 poles (53.7276, 63.4965) (51.7915, 63.4965) (51.155, 65.026) (51.155, 67.0072) knots 0 0 0 0 1 1 1 1
  line L317 (51.155, 67.0072) -> (51.155, 70.1829)
  line L318 (51.155, 70.1829) -> (59.8276, 70.1828)
  line L319 (55.2128, 68.493) -> (52.3883, 68.493)
  line L320 (52.3883, 68.493) -> (52.3883, 67.182)
  spline S72 degree 3 poles (52.3883, 67.182) (52.3883, 65.8709) (52.733, 65.1571) (53.7276, 65.1571) knots 0 0 0 0 1 1 1 1
  spline S73 degree 3 poles (53.7276, 65.1571) (54.7089, 65.1571) (55.2128, 65.8709) (55.2128, 67.182) knots 0 0 0 0 1 1 1 1
  line L321 (55.2128, 67.182) -> (55.2128, 68.493)
  line L322 (59.8276, 50.4119) -> (59.8276, 48.7221)
  line L323 (59.8276, 48.7221) -> (52.4546, 48.7221)
  line L324 (52.4546, 48.7221) -> (52.4546, 45.7212)
  line L325 (52.4546, 45.7212) -> (51.155, 45.7212)
  line L326 (51.155, 45.7212) -> (51.155, 53.4128)
  line L327 (51.155, 53.4128) -> (52.4546, 53.4128)
  line L328 (52.4546, 53.4128) -> (52.4546, 50.4119)
  line L329 (52.4546, 50.4119) -> (59.8276, 50.4119)
  line L330 (59.8276, 34.9674) -> (59.8276, 28.718)
  line L331 (59.8276, 28.718) -> (58.528, 28.718)
  line L332 (58.528, 28.718) -> (58.528, 33.2775)
  line L333 (58.528, 33.2775) -> (55.9687, 33.2775)
  line L334 (55.9687, 33.2775) -> (55.9687, 29.5337)
  line L335 (55.9687, 29.5337) -> (54.6691, 29.5337)
  line L336 (54.6691, 29.5337) -> (54.6691, 33.2775)
  line L337 (54.6691, 33.2775) -> (52.4545, 33.2775)
  line L338 (52.4545, 33.2775) -> (52.4545, 28.8637)
  line L339 (52.4545, 28.8637) -> (51.155, 28.8637)
  line L340 (51.155, 28.8637) -> (51.155, 34.9674)
  line L341 (51.155, 34.9674) -> (59.8276, 34.9674)
  line L342 (59.8276, 17.2504) -> (59.8276, 11.103)
  line L343 (59.8276, 11.103) -> (58.528, 11.103)
  line L344 (58.528, 11.103) -> (58.528, 15.5752)
  line L345 (58.528, 15.5752) -> (51.155, 15.5752)
  line L346 (51.155, 15.5752) -> (51.155, 17.2504)
  line L347 (51.155, 17.2504) -> (59.8276, 17.2504)
  line L348 (78.8701, 190.3123) -> (78.8701, 188.3166)
  line L349 (78.8701, 188.3166) -> (70.1975, 185.3594)
  line L350 (70.1975, 185.3594) -> (70.1975, 187.0929)
  line L351 (70.1975, 187.0929) -> (74.5603, 188.4185)
  spline S74 degree 3 poles (74.5603, 188.4185) (75.5416, 188.7099) (76.3903, 188.9284) (77.3849, 189.2489) knots 0 0 0 0 1 1 1 1
  line L352 (77.3849, 189.2489) -> (77.3849, 189.3071)
  spline S75 degree 3 poles (77.3849, 189.3071) (76.3903, 189.6276) (75.5416, 189.8461) (74.5603, 190.152) knots 0 0 0 0 1 1 1 1
  line L353 (74.5603, 190.152) -> (70.1975, 191.4922)
  line L354 (70.1975, 191.4922) -> (70.1975, 193.284)
  line L355 (70.1975, 193.284) -> (78.8701, 190.3123)
  spline S76 degree 3 poles (79.0292, 171.8524) (79.0292, 169.6381) (77.3981, 168.1086) (74.494, 168.1086) knots 0 0 0 0 1 1 1 1
  spline S77 degree 3 poles (74.494, 168.1086) (71.6429, 168.1086) (70.0384, 169.6381) (70.0384, 171.8524) knots 0 0 0 0 1 1 1 1
  spline S78 degree 3 poles (70.0384, 171.8524) (70.0384, 174.0666) (71.6429, 175.5962) (74.494, 175.5962) knots 0 0 0 0 1 1 1 1
  spline S79 degree 3 poles (74.494, 175.5962) (77.3981, 175.5962) (79.0292, 174.0666) (79.0292, 171.8524) knots 0 0 0 0 1 1 1 1
  spline S80 degree 3 poles (77.6899, 171.8524) (77.6899, 173.076) (76.5362, 173.8626) (74.494, 173.8626) knots 0 0 0 0 1 1 1 1
  spline S81 degree 3 poles (74.494, 173.8626) (72.5049, 173.8626) (71.3777, 173.076) (71.3777, 171.8524) knots 0 0 0 0 1 1 1 1
  spline S82 degree 3 poles (71.3777, 171.8524) (71.3777, 170.6287) (72.5049, 169.8421) (74.494, 169.8421) knots 0 0 0 0 1 1 1 1
  spline S83 degree 3 poles (74.494, 169.8421) (76.5362, 169.8421) (77.6899, 170.6287) (77.6899, 171.8524) knots 0 0 0 0 1 1 1 1
  line L356 (78.8701, 157.5296) -> (78.8701, 155.8398)
  line L357 (78.8701, 155.8398) -> (75.4753, 155.8398)
  line L358 (75.4753, 155.8398) -> (75.4753, 154.4122)
  line L359 (75.4753, 154.4122) -> (78.8701, 152.3728)
  line L360 (78.8701, 152.3728) -> (78.8701, 150.4644)
  line L361 (78.8701, 150.4644) -> (75.2499, 152.7369)
  spline S84 degree 3 poles (75.2499, 152.7369) (74.8918, 151.6007) (74.0829, 150.8432) (72.7701, 150.8432) knots 0 0 0 0 1 1 1 1
  spline S85 degree 3 poles (72.7701, 150.8432) (70.834, 150.8432) (70.1975, 152.3728) (70.1975, 154.3539) knots 0 0 0 0 1 1 1 1
  line L362 (70.1975, 154.3539) -> (70.1975, 157.5296)
  line L363 (70.1975, 157.5296) -> (78.8701, 157.5296)
  line L364 (74.2553, 155.8398) -> (71.4307, 155.8398)
  line L365 (71.4307, 155.8398) -> (71.4307, 154.5287)
  spline S86 degree 3 poles (71.4307, 154.5287) (71.4307, 153.2177) (71.7755, 152.5039) (72.7701, 152.5039) knots 0 0 0 0 1 1 1 1
  spline S87 degree 3 poles (72.7701, 152.5039) (73.7514, 152.5039) (74.2553, 153.2177) (74.2553, 154.5287) knots 0 0 0 0 1 1 1 1
  line L366 (74.2553, 154.5287) -> (74.2553, 155.8398)
  line L367 (78.8701, 139.5504) -> (78.8701, 137.8605)
  line L368 (78.8701, 137.8605) -> (75.2499, 137.8605)
  line L369 (75.2499, 137.8605) -> (75.2499, 134.1168)
  line L370 (75.2499, 134.1168) -> (73.9503, 134.1168)
  line L371 (73.9503, 134.1168) -> (73.9503, 137.8605)
  line L372 (73.9503, 137.8605) -> (71.4971, 137.8605)
  line L373 (71.4971, 137.8605) -> (71.4971, 133.4612)
  line L374 (71.4971, 133.4612) -> (70.1975, 133.4612)
  line L375 (70.1975, 133.4612) -> (70.1975, 139.5504)
  line L376 (70.1975, 139.5504) -> (78.8701, 139.5504)
  spline S88 degree 3 poles (79.0292, 119.4298) (79.0292, 117.3321) (77.9286, 116.123) (75.5549, 116.123) knots 0 0 0 0 1 1 1 1
  line L377 (75.5549, 116.123) -> (70.1975, 116.123)
  line L378 (70.1975, 116.123) -> (70.1975, 117.74)
  line L379 (70.1975, 117.74) -> (75.6742, 117.74)
  spline S89 degree 3 poles (75.6742, 117.74) (77.0931, 117.74) (77.6899, 118.3955) (77.6899, 119.4297) knots 0 0 0 0 1 1 1 1
  spline S90 degree 3 poles (77.6899, 119.4297) (77.6899, 120.4495) (77.0931, 121.0759) (75.6742, 121.0759) knots 0 0 0 0 1 1 1 1
  line L380 (75.6742, 121.0759) -> (70.1975, 121.0759)
  line L381 (70.1975, 121.0759) -> (70.1975, 122.7656)
  line L382 (70.1975, 122.7656) -> (75.5549, 122.7656)
  spline S91 degree 3 poles (75.5549, 122.7656) (77.9286, 122.7656) (79.0292, 121.5129) (79.0292, 119.4298) knots 0 0 0 0 1 1 1 1
  line L383 (78.8701, 105.2672) -> (78.8701, 103.6502)
  line L384 (78.8701, 103.6502) -> (75.0775, 103.6502)
  spline S92 degree 3 poles (75.0775, 103.6502) (74.1094, 103.6502) (73.0751, 103.8105) (72.1468, 103.8833) knots 0 0 0 0 1 1 1 1
  line L385 (72.1468, 103.8833) -> (72.1468, 103.8396)
  line L386 (72.1468, 103.8396) -> (73.9901, 102.9801)
  line L387 (73.9901, 102.9801) -> (78.8701, 100.46)
  line L388 (78.8701, 100.46) -> (78.8701, 98.6828)
  line L389 (78.8701, 98.6828) -> (70.1975, 98.6828)
  line L390 (70.1975, 98.6828) -> (70.1975, 100.2997)
  line L391 (70.1975, 100.2997) -> (73.9636, 100.2997)
  spline S93 degree 3 poles (73.9636, 100.2997) (74.9316, 100.2997) (76.0323, 100.1395) (76.9207, 100.0667) knots 0 0 0 0 1 1 1 1
  line L392 (76.9207, 100.0667) -> (76.9207, 100.1104)
  line L393 (76.9207, 100.1104) -> (75.0642, 100.9699)
  line L394 (75.0642, 100.9699) -> (70.1975, 103.49)
  line L395 (70.1975, 103.49) -> (70.1975, 105.2672)
  line L396 (70.1975, 105.2672) -> (78.8701, 105.2672)
  line L397 (78.8701, 87.6813) -> (78.8701, 85.9624)
  line L398 (78.8701, 85.9624) -> (76.3107, 85.9624)
  line L399 (76.3107, 85.9624) -> (74.746, 84.6076)
  line L400 (74.746, 84.6076) -> (78.8701, 82.204)
  line L401 (78.8701, 82.204) -> (78.8701, 80.3248)
  line L402 (78.8701, 80.3248) -> (73.5657, 83.5733)
  line L403 (73.5657, 83.5733) -> (70.1975, 80.6308)
  line L404 (70.1975, 80.6308) -> (70.1975, 82.5245)
  line L405 (70.1975, 82.5245) -> (74.1359, 85.9187)
  line L406 (74.1359, 85.9187) -> (74.1359, 85.9624)
  line L407 (74.1359, 85.9624) -> (70.1975, 85.9624)
  line L408 (70.1975, 85.9624) -> (70.1975, 87.6813)
  line L409 (70.1975, 87.6813) -> (78.8701, 87.6813)
  line L410 (78.8701, 70.3285) -> (78.8701, 68.7116)
  line L411 (78.8701, 68.7116) -> (75.0775, 68.7116)
  spline S94 degree 3 poles (75.0775, 68.7116) (74.1094, 68.7116) (73.0751, 68.8718) (72.1468, 68.9446) knots 0 0 0 0 1 1 1 1
  line L412 (72.1468, 68.9446) -> (72.1468, 68.9009)
  line L413 (72.1468, 68.9009) -> (73.9901, 68.0415)
  line L414 (73.9901, 68.0415) -> (78.8701, 65.5213)
  line L415 (78.8701, 65.5213) -> (78.8701, 63.7441)
  line L416 (78.8701, 63.7441) -> (70.1975, 63.7441)
  line L417 (70.1975, 63.7441) -> (70.1975, 65.3611)
  line L418 (70.1975, 65.3611) -> (73.9636, 65.3611)
  spline S95 degree 3 poles (73.9636, 65.3611) (74.9316, 65.3611) (76.0323, 65.2008) (76.9207, 65.128) knots 0 0 0 0 1 1 1 1
  line L419 (76.9207, 65.128) -> (76.9207, 65.1717)
  line L420 (76.9207, 65.1717) -> (75.0642, 66.0312)
  line L421 (75.0642, 66.0312) -> (70.1975, 68.5513)
  line L422 (70.1975, 68.5513) -> (70.1975, 70.3285)
  line L423 (70.1975, 70.3285) -> (78.8701, 70.3285)
  spline S96 degree 3 poles (74.2553, 50.4701) (73.3403, 50.1788) (72.359, 49.8875) (71.391, 49.6252) knots 0 0 0 0 1 1 1 1
  line L424 (71.391, 49.6252) -> (71.391, 49.567)
  spline S97 degree 3 poles (71.391, 49.567) (72.359, 49.3048) (73.3403, 48.9989) (74.2553, 48.7221) knots 0 0 0 0 1 1 1 1
  line L425 (74.2553, 48.7221) -> (75.3162, 48.387)
  line L426 (75.3162, 48.387) -> (75.3162, 50.8052)
  line L427 (75.3162, 50.8052) -> (74.2553, 50.4701)
  line L428 (78.8701, 53.6458) -> (78.8701, 51.9269)
  line L429 (78.8701, 51.9269) -> (76.5229, 51.1839)
  line L430 (76.5229, 51.1839) -> (76.5229, 48.0083)
  line L431 (76.5229, 48.0083) -> (78.8701, 47.2799)
  line L432 (78.8701, 47.2799) -> (78.8701, 45.4881)
  line L433 (78.8701, 45.4881) -> (70.1975, 48.5764)
  line L434 (70.1975, 48.5764) -> (70.1975, 50.5576)
  line L435 (70.1975, 50.5576) -> (78.8701, 53.6458)
  spline S98 degree 3 poles (79.0292, 31.311) (79.0292, 30.0436) (78.5783, 29.0385) (77.7694, 28.281) knots 0 0 0 0 1 1 1 1
  line L436 (77.7694, 28.281) -> (76.8279, 29.2133)
  spline S99 degree 3 poles (76.8279, 29.2133) (77.3716, 29.7523) (77.6899, 30.3787) (77.6899, 31.1508) knots 0 0 0 0 1 1 1 1
  spline S100 degree 3 poles (77.6899, 31.1508) (77.6899, 32.7823) (76.4964, 33.8603) (74.5205, 33.8603) knots 0 0 0 0 1 1 1 1
  spline S101 degree 3 poles (74.5205, 33.8603) (72.5712, 33.8603) (71.3777, 32.7823) (71.3777, 31.1945) knots 0 0 0 0 1 1 1 1
  spline S102 degree 3 poles (71.3777, 31.1945) (71.3777, 30.4516) (71.6562, 29.8834) (72.0805, 29.4027) knots 0 0 0 0 1 1 1 1
  line L437 (72.0805, 29.4027) -> (71.1257, 28.4704)
  spline S103 degree 3 poles (71.1257, 28.4704) (70.5555, 29.0676) (70.0384, 30.0145) (70.0384, 31.1945) knots 0 0 0 0 1 1 1 1
  spline S104 degree 3 poles (70.0384, 31.1945) (70.0384, 33.7146) (71.7225, 35.5938) (74.5603, 35.5938) knots 0 0 0 0 1 1 1 1
  spline S105 degree 3 poles (74.5603, 35.5938) (77.4379, 35.5938) (79.0292, 33.6709) (79.0292, 31.311) knots 0 0 0 0 1 1 1 1
  line L438 (78.8701, 17.9496) -> (78.8701, 16.2598)
  line L439 (78.8701, 16.2598) -> (75.0244, 16.2598)
  line L440 (75.0244, 16.2598) -> (75.0244, 12.9967)
  line L441 (75.0244, 12.9967) -> (78.8701, 12.9967)
  line L442 (78.8701, 12.9967) -> (78.8701, 11.3069)
  line L443 (78.8701, 11.3069) -> (70.1975, 11.3069)
  line L444 (70.1975, 11.3069) -> (70.1975, 12.9967)
  line L445 (70.1975, 12.9967) -> (73.6851, 12.9967)
  line L446 (73.6851, 12.9967) -> (73.6851, 16.2598)
  line L447 (73.6851, 16.2598) -> (70.1975, 16.2598)
  line L448 (70.1975, 16.2598) -> (70.1975, 17.9496)
  line L449 (70.1975, 17.9496) -> (78.8701, 17.9496)
  line L450 (97.9126, 192.643) -> (97.9126, 190.9532)
  line L451 (97.9126, 190.9532) -> (94.0669, 190.9532)
  line L452 (94.0669, 190.9532) -> (94.0669, 187.6902)
  line L453 (94.0669, 187.6902) -> (97.9126, 187.6902)
  line L454 (97.9126, 187.6902) -> (97.9126, 186.0004)
  line L455 (97.9126, 186.0004) -> (89.24, 186.0004)
  line L456 (89.24, 186.0004) -> (89.24, 187.6902)
  line L457 (89.24, 187.6902) -> (92.7276, 187.6902)
  line L458 (92.7276, 187.6902) -> (92.7276, 190.9532)
  line L459 (92.7276, 190.9532) -> (89.24, 190.9532)
  line L460 (89.24, 190.9532) -> (89.24, 192.643)
  line L461 (89.24, 192.643) -> (97.9126, 192.643)
  spline S106 degree 3 poles (93.2978, 172.7555) (92.3828, 172.4642) (91.4015, 172.1729) (90.4335, 171.9106) knots 0 0 0 0 1 1 1 1
  line L462 (90.4335, 171.9106) -> (90.4335, 171.8524)
  spline S107 degree 3 poles (90.4335, 171.8524) (91.4015, 171.5902) (92.3828, 171.2843) (93.2978, 171.0075) knots 0 0 0 0 1 1 1 1
  line L463 (93.2978, 171.0075) -> (94.3587, 170.6724)
  line L464 (94.3587, 170.6724) -> (94.3587, 173.0906)
  line L465 (94.3587, 173.0906) -> (93.2978, 172.7555)
  line L466 (97.9126, 175.9312) -> (97.9126, 174.2123)
  line L467 (97.9126, 174.2123) -> (95.5654, 173.4693)
  line L468 (95.5654, 173.4693) -> (95.5654, 170.2937)
  line L469 (95.5654, 170.2937) -> (97.9126, 169.5653)
  line L470 (97.9126, 169.5653) -> (97.9126, 167.7735)
  line L471 (97.9126, 167.7735) -> (89.24, 170.8618)
  line L472 (89.24, 170.8618) -> (89.24, 172.8429)
  line L473 (89.24, 172.8429) -> (97.9126, 175.9312)
  line L474 (97.9126, 157.0051) -> (97.9126, 150.8577)
  line L475 (97.9126, 150.8577) -> (96.613, 150.8577)
  line L476 (96.613, 150.8577) -> (96.613, 155.3299)
  line L477 (96.613, 155.3299) -> (89.24, 155.3299)
  line L478 (89.24, 155.3299) -> (89.24, 157.0051)
  line L479 (89.24, 157.0051) -> (97.9126, 157.0051)
  line L480 (97.9126, 140.0311) -> (97.9126, 136.8263)
  spline S108 degree 3 poles (97.9126, 136.8263) (97.9126, 134.7286) (97.1037, 133.199) (95.3665, 133.199) knots 0 0 0 0 1 1 1 1
  spline S109 degree 3 poles (95.3665, 133.199) (94.1863, 133.199) (93.5232, 133.9711) (93.3111, 135.3404) knots 0 0 0 0 1 1 1 1
  line L481 (93.3111, 135.3404) -> (93.258, 135.3404)
  spline S110 degree 3 poles (93.258, 135.3404) (92.9928, 134.2187) (92.1971, 133.6943) (91.375, 133.6943) knots 0 0 0 0 1 1 1 1
  spline S111 degree 3 poles (91.375, 133.6943) (89.7837, 133.6943) (89.24, 135.1074) (89.24, 137.0739) knots 0 0 0 0 1 1 1 1
  line L482 (89.24, 137.0739) -> (89.24, 140.0311)
  line L483 (89.24, 140.0311) -> (97.9126, 140.0311)
  line L484 (92.8071, 138.3413) -> (90.4732, 138.3413)
  line L485 (90.4732, 138.3413) -> (90.4732, 137.1905)
  spline S112 degree 3 poles (90.4732, 137.1905) (90.4732, 135.9522) (90.765, 135.355) (91.5606, 135.355) knots 0 0 0 0 1 1 1 1
  spline S113 degree 3 poles (91.5606, 135.355) (92.3695, 135.355) (92.8071, 135.894) (92.8071, 137.2196) knots 0 0 0 0 1 1 1 1
  line L486 (92.8071, 137.2196) -> (92.8071, 138.3413)
  line L487 (96.6793, 138.3413) -> (93.9741, 138.3413)
  line L488 (93.9741, 138.3413) -> (93.9741, 137.0011)
  spline S114 degree 3 poles (93.9741, 137.0011) (93.9741, 135.5735) (94.3454, 134.8597) (95.2604, 134.8597) knots 0 0 0 0 1 1 1 1
  spline S115 degree 3 poles (95.2604, 134.8597) (96.2417, 134.8597) (96.6793, 135.6026) (96.6793, 137.0011) knots 0 0 0 0 1 1 1 1
  line L489 (96.6793, 137.0011) -> (96.6793, 138.3413)
  spline S116 degree 3 poles (93.2978, 120.3475) (92.3828, 120.0562) (91.4015, 119.7648) (90.4335, 119.5026) knots 0 0 0 0 1 1 1 1
  line L490 (90.4335, 119.5026) -> (90.4335, 119.4443)
  spline S117 degree 3 poles (90.4335, 119.4443) (91.4015, 119.1821) (92.3828, 118.8762) (93.2978, 118.5994) knots 0 0 0 0 1 1 1 1
  line L491 (93.2978, 118.5994) -> (94.3587, 118.2644)
  line L492 (94.3587, 118.2644) -> (94.3587, 120.6825)
  line L493 (94.3587, 120.6825) -> (93.2978, 120.3475)
  line L494 (97.9126, 123.5232) -> (97.9126, 121.8042)
  line L495 (97.9126, 121.8042) -> (95.5654, 121.0613)
  line L496 (95.5654, 121.0613) -> (95.5654, 117.8856)
  line L497 (95.5654, 117.8856) -> (97.9126, 117.1573)
  line L498 (97.9126, 117.1573) -> (97.9126, 115.3655)
  line L499 (97.9126, 115.3655) -> (89.24, 118.4538)
  line L500 (89.24, 118.4538) -> (89.24, 120.4349)
  line L501 (89.24, 120.4349) -> (97.9126, 123.5232)
  line L502 (97.9126, 104.8447) -> (97.9126, 98.5954)
  line L503 (97.9126, 98.5954) -> (96.613, 98.5954)
  line L504 (96.613, 98.5954) -> (96.613, 103.155)
  line L505 (96.613, 103.155) -> (94.0537, 103.155)
  line L506 (94.0537, 103.155) -> (94.0537, 99.4112)
  line L507 (94.0537, 99.4112) -> (92.7541, 99.4112)
  line L508 (92.7541, 99.4112) -> (92.7541, 103.155)
  line L509 (92.7541, 103.155) -> (90.5395, 103.155)
  line L510 (90.5395, 103.155) -> (90.5395, 98.7411)
  line L511 (90.5395, 98.7411) -> (89.24, 98.7411)
  line L512 (89.24, 98.7411) -> (89.24, 104.8447)
  line L513 (89.24, 104.8447) -> (97.9126, 104.8447)
  line L514 (97.9126, 87.1278) -> (97.9126, 80.9804)
  line L515 (97.9126, 80.9804) -> (96.613, 80.9804)
  line L516 (96.613, 80.9804) -> (96.613, 85.4525)
  line L517 (96.613, 85.4525) -> (89.24, 85.4525)
  line L518 (89.24, 85.4525) -> (89.24, 87.1278)
  line L519 (89.24, 87.1278) -> (97.9126, 87.1278)
  line L520 (97.9126, 69.673) -> (97.9126, 67.9832)
  line L521 (97.9126, 67.9832) -> (94.2924, 67.9832)
  line L522 (94.2924, 67.9832) -> (94.2924, 64.2394)
  line L523 (94.2924, 64.2394) -> (92.9928, 64.2394)
  line L524 (92.9928, 64.2394) -> (92.9928, 67.9832)
  line L525 (92.9928, 67.9832) -> (90.5396, 67.9832)
  line L526 (90.5396, 67.9832) -> (90.5396, 63.5839)
  line L527 (90.5396, 63.5839) -> (89.24, 63.5839)
  line L528 (89.24, 63.5839) -> (89.24, 69.673)
  line L529 (89.24, 69.673) -> (97.9126, 69.673)
  spline S118 degree 3 poles (98.0717, 49.5524) (98.0717, 47.4547) (96.9711, 46.2456) (94.5973, 46.2456) knots 0 0 0 0 1 1 1 1
  line L530 (94.5973, 46.2456) -> (89.24, 46.2456)
  line L531 (89.24, 46.2456) -> (89.24, 47.8626)
  line L532 (89.24, 47.8626) -> (94.7167, 47.8626)
  spline S119 degree 3 poles (94.7167, 47.8626) (96.1356, 47.8626) (96.7323, 48.5181) (96.7323, 49.5524) knots 0 0 0 0 1 1 1 1
  spline S120 degree 3 poles (96.7323, 49.5524) (96.7323, 50.5721) (96.1356, 51.1985) (94.7167, 51.1985) knots 0 0 0 0 1 1 1 1